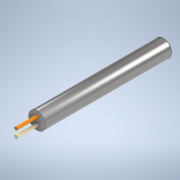
# Autodesk Inventor part: HP_8x60_160W
Saved by Autodesk Inventor 2021 (Build 250183000, 183)
## iProperties
Created: 2021-05-06
Part Number: HP_8x60_160W
Material: Edelstahl, 440C
Document SubType Name: Modeling
Designer: Sebastian Seewald
Mass: 23.3633 g
Surface Area: 16.0299 cm^2
Volume: 3.01462 cm^3
Density: 7.75 g/cm^3
Appearance: Halbpoliert
Author: Sebastian Seewald
Autodesk Inventor part; units mm, degrees
ref_plane "YZ Plane" through (0, 0, 0) normal (1, 0, 0) x (0, 1, 0)
ref_plane "XZ Plane" through (0, 0, 0) normal (0, 1, 0) x (-1, 0, 0)
ref_plane "XY Plane" through (0, 0, 0) normal (0, 0, 1) x (1, 0, 0)
sketch "Skizze1" plane through (0, 0, 0) normal (0, 0, 1) x (1, 0, 0)
  circle A0 centre (0, 0) radius 4
  dimension "d0" = 8
  constraints: 1 centre point, 1 coincident
  measures "d0" diameter of A0
extrude "Extrusion1" add sketch "Skizze1" along normal blind 60
fillet "Rundung1" radius 0.5 1 edges at (-4, 0, 0)
sketch "Skizze2" plane through (0, 0, 60) normal (0, 0, 1) x (1, 0, 0)
  circle A0 centre (0, 1.7) radius 0.65
  circle A1 centre (0, -1.7) radius 0.65
  point P0 (0, 0)
  dimension "d4" = 1.3
  dimension "d5" = 1.3
  dimension "d6" = 1.7
  dimension "d7" = 1.7
  constraints: 2 centre point
  measures "d4" diameter of A1
  measures "d5" diameter of A0
  measures "d6" distance of point (0, 0) A0.centre
  measures "d7" distance of point (0, 0) A1.centre
extrude "Extrusion2" add sketch "Skizze2" along normal blind 10
sketch "Skizze3" plane through (0, 1.7, 70) normal (0, 0, 1) x (1, 0, 0)
  point P0 (0, -1.7)
